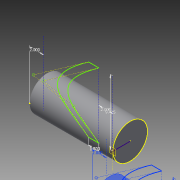
# Autodesk Inventor part: Drum
Saved by Autodesk Inventor 2015 (Build 190159000, 159)
## iProperties
Created: 2015-04-20
Part Number: Drum
Material: Generic
Document SubType Name: Modeling
Designer: WASHHSST
Density: 1 g/cm^3
Appearance: Default
Author: WASHHSST
Autodesk Inventor part; units mm, degrees
ref_plane "YZ Plane" through (0, 0, 0) normal (1, 0, 0) x (0, 1, 0)
ref_plane "XZ Plane" through (0, 0, 0) normal (0, 1, 0) x (-1, 0, 0)
ref_plane "XY Plane" through (0, 0, 0) normal (0, 0, 1) x (1, 0, 0)
sketch "Sketch1" plane through (0, 0, 0) normal (1, 0, 0) x (0, 1, 0)
  circle A0 centre (0, 0) radius 63.5
  dimension "d0" = 127
  constraints: 1 centre point, 1 coincident
  measures "d0" diameter of A0
extrude "Extrusion1" add sketch "Sketch1" along normal blind 304.8
sketch "Sketch2" plane through (304.8, 0, 0) normal (1, 0, 0) x (0, 0, -1)
  line L0 (0, 0) -> (-63.5, 0)
  circle A0 centre (0, 0) radius 63.5 projected
  constraints: 2 end point, 1 horizontal, 1 horizontal alignment, 1 other
ref_plane "Work Plane1" through (304.8, 0, 63.5) normal (0, 0, 1) x (1, 0, 0)
sketch "Sketch4" plane through (304.8, 0, 63.5) normal (0, 0, 1) x (1, 0, 0)
  line L0 (0, -63.5) -> (0, 63.5) construction
  line L1 (0, 0) -> (0, 239.3894) construction
  line L2 (-50.8, 0) -> (-50.8, 239.3894) construction
  line L3 (-254, 0) -> (-254, 239.3894) construction
  line L4 (-50.8, 0) -> (-143.4153, 70.3949) construction
  line L5 (-143.4153, 70.3949) -> (-254, 96.3991) construction
  line L6 (-254, 96.3991) -> (-50.8, 239.3894) construction
  spline S0 degree 3 poles (-50.8, 0) (-143.4153, 70.3949) (-254, 96.3991) (-50.8, 239.3894) knots 1 1 1 1 2 2 2 2
  line L7 (-88.9, 0) -> (-181.5153, 70.3949) construction
  line L8 (-181.5153, 70.3949) -> (-292.1, 96.3991) construction
  line L9 (-292.1, 96.3991) -> (-88.9, 239.3894) construction
  spline S1 degree 3 poles (-88.9, 0) (-181.5153, 70.3949) (-292.1, 96.3991) (-88.9, 239.3894) knots 1 1 1 1 2 2 2 2
  line L10 (-88.9, 0) -> (-50.8, 0)
  line L11 (-88.9, 239.3894) -> (-50.8, 239.3894)
  point P0 (-304.8, 0)
  dimension "d5" = 239.3894
  dimension "d6" = 50.8
  dimension "d7" = 50.8
  dimension "d8" = 38.1
  constraints: 10 end point, 3 parallel, 1 collinear, 1 horizontal, 1 midpoint, 1 point on line, 6 other
  measures "d5" distance of L1.start L1.end
  measures "d6" distance between parallel lines of L1 L2
  measures "d7" distance from line of point (-304.8, 0) L3
  measures "d8" distance of L2.start L7.start
body "Solid1"
